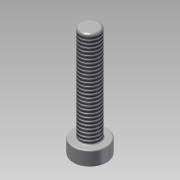
# Autodesk Inventor part: Vis-Pivot
Saved by Autodesk Inventor 2016 (Build 200138000, 138)
## iProperties
Created: 2016-01-27
Part Number: Vis-Pivot
Material: Acier
Document SubType Name: Modeling
Designer: sd
Density: 7.85 g/cm^3
Appearance: Acier
Mass: 2.81147 g
Surface Area: 3.95632 cm^2
Volume: 0.358149 cm^3
Author: sd
Autodesk Inventor part; units mm, degrees
ref_plane "YZ Plane" through (0, 0, 0) normal (1, 0, 0) x (0, 1, 0)
ref_plane "XZ Plane" through (0, 0, 0) normal (0, 1, 0) x (-1, 0, 0)
ref_plane "XY Plane" through (0, 0, 0) normal (0, 0, 1) x (1, 0, 0)
sketch "Esquisse1" plane through (0, 0, 0) normal (0, 0, 1) x (1, 0, 0)
  circle A0 centre (0, 0) radius 3.5
  dimension "d0" = 7
  constraints: 1 centre point, 1 coincident
  measures "d0" diameter of A0
extrude "Extrusion1" add sketch "Esquisse1" along normal blind 3
sketch "Esquisse2" plane through (0, 0, 3) normal (0, 0, 1) x (1, 0, 0)
  circle A0 centre (0, 0) radius 3.5 projected
  circle A1 centre (0, 0) radius 2
  dimension "d3" = 4
  constraints: 1 centre point, 1 coincident
  measures "d3" diameter of A1
extrude "Extrusion2" add sketch "Esquisse2" along normal blind 20 contours A1
fillet "Congé1" radius 0.5 1 edges at (-2, 0, 23)
thread "Filetage1" size "M4x0.7" class "6g" standard "ANSI Metric M Profile" full length
fillet "Congé2" radius 0.25 2 edges at (-3.5, 0, 0) (-3.5, 0, 3)
sketch "Esquisse3" plane through (0, 0, 0) normal (0, 0, -1) x (-1, 0, 0)
  circle A0 centre (0, 0) radius 3.25 projected
  line L0 (0, 1.4434) -> (1.25, 0.7217)
  line L1 (1.25, 0.7217) -> (1.25, -0.7217)
  line L2 (1.25, -0.7217) -> (0, -1.4434)
  line L3 (0, -1.4434) -> (-1.25, -0.7217)
  line L4 (-1.25, -0.7217) -> (-1.25, 0.7217)
  line L5 (-1.25, 0.7217) -> (0, 1.4434)
  dimension "d10" = 2.5
  constraints: 12 end point, 1 coincident, 13 other
  measures "d10" distance between parallel lines of L1 L4
extrude "Extrusion3" cut sketch "Esquisse3" against normal blind 1.4 contours L0 L1 L2 L3 L4 L5
fillet "Congé3" radius 0.25 12 edges at (-0.625, 1.0825, 0) (-1.25, 0, 0) (-0.625, -1.0825, 0) (0.625, -1.0825, 0) (1.25, 0, 0) (0.625, 1.0825, 0) (-0.625, 1.0825, 1.4) (0.625, 1.0825, 1.4) (1.25, 0, 1.4) (0.625, -1.0825, 1.4) (-0.625, -1.0825, 1.4) (-1.25, 0, 1.4)
fillet "Congé4" radius 0.25 1 edges at (-2, 0, 3)
